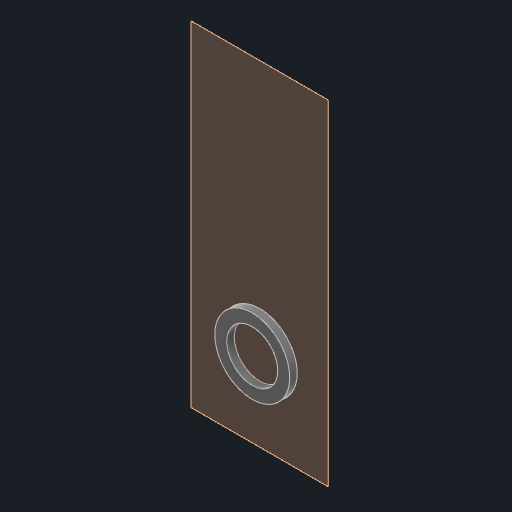
# Autodesk Inventor part: Ubber_Washer_1.5mm
Saved by Autodesk Inventor 2024 (Build 280153000, 153)
## iProperties
Created: 2024-01-25
Part Number: Ubber_Washer_1.5mm
Material: LCP 플라스틱
Document SubType Name: Modeling
Designer: ASUS
Density: 1.626 g/cm^3
Appearance: 매끄러움 - 검은색
Author: ASUS
Autodesk Inventor part; units mm, degrees
ref_plane "YZ Plane" through (0, 0, 0) normal (1, 0, 0) x (0, 1, 0)
ref_plane "XZ Plane" through (0, 0, 0) normal (0, 1, 0) x (-1, 0, 0)
ref_plane "XY Plane" through (0, 0, 0) normal (0, 0, 1) x (1, 0, 0)
ref_plane "작업 평면1" through (0, 0, 0) normal (0, 0, 1) x (1, 0, 0)
sketch "스케치1" plane through (0, 0, 0) normal (0, 0, 1) x (1, 0, 0)
  circle A0 centre (-3, -27.5) radius 1.35 projected
  circle A1 centre (3, -27.5) radius 1.35 projected
  line L0 (4.4, -3.4094) -> (4.4, -19.8749) projected
  arc A2 (-4.4, -19.8749) -> (4.4, -19.8749) centre (0, -17.5) ccw projected
  line L1 (-4.4, -19.8749) -> (-4.4, -3.4094) projected
  arc A3 (4.4, -3.4094) -> (-4.4, -3.4094) centre (0, -5.7843) ccw projected
  circle A4 centre (0, 22.5) radius 4 projected
  arc A5 (-2.7698, 16.0713) -> (2.7698, 16.0713) centre (0, 22.5) ccw projected
  arc A6 (5.5454, 14.4845) -> (2.7698, 16.0713) centre (3.5611, 14.2345) ccw projected
  line L2 (5.5454, 14.4845) -> (6.9428, 3.3933) projected
  arc A7 (3.9674, 1.4062) -> (6.9428, 3.3933) centre (4.9585, 3.1433) ccw projected
  arc A8 (3.9674, 1.4062) -> (-3.9674, 1.4062) centre (0, -5.5476) ccw projected
  arc A9 (-6.9428, 3.3933) -> (-3.9674, 1.4062) centre (-4.9585, 3.1433) ccw projected
  line L3 (-6.9428, 3.3933) -> (-5.5454, 14.4845) projected
  arc A10 (-2.7698, 16.0713) -> (-5.5454, 14.4845) centre (-3.5611, 14.2345) ccw projected
  arc A11 (-12.5, -19.9495) -> (-9.6429, -26.948) centre (-2.5, -19.9495) ccw projected
  arc A12 (-9.6429, -26.948) -> (9.6429, -26.948) centre (0, -17.5) ccw projected
  arc A13 (9.6429, -26.948) -> (12.5, -19.9495) centre (2.5, -19.9495) ccw projected
  line L4 (12.5, -19.9495) -> (12.5, -17.5) projected
  arc A14 (12.5, -17.5) -> (12.402, -15.9375) centre (0, -17.5) ccw projected
  line L5 (7.4412, 23.4375) -> (12.402, -15.9375) projected
  arc A15 (7.4412, 23.4375) -> (-7.4412, 23.4375) centre (0, 22.5) ccw projected
  line L6 (-12.402, -15.9375) -> (-7.4412, 23.4375) projected
  arc A16 (-12.402, -15.9375) -> (-12.5, -17.5) centre (0, -17.5) ccw projected
  line L7 (-12.5, -17.5) -> (-12.5, -19.9495) projected
  circle A17 centre (0, -17.5) radius 3 projected
  line L8 (-4.4, -16.5566) -> (-4.4, -18.4434) projected
  arc A18 (-4.4, -18.4434) -> (4.4, -18.4434) centre (0, -17.5) ccw projected
  line L9 (4.4, -18.4434) -> (4.4, -16.5566) projected
  arc A19 (4.4, -16.5566) -> (-4.4, -16.5566) centre (0, -17.5) ccw projected
  circle A20 centre (0, -17.5) radius 5.1
  circle A21 centre (0, -17.5) radius 7.5
  point P0 (0, 0)
  dimension "d0" = 10.2
  dimension "d1" = 15
  constraints: 2 centre point, 2 coincident
  measures "d0" diameter of A20
  measures "d1" diameter of A21
extrude "돌출1" add sketch "스케치1" along normal blind 1.5 contours A20 L1 A21 L0 | L0 A21 L1 A20
